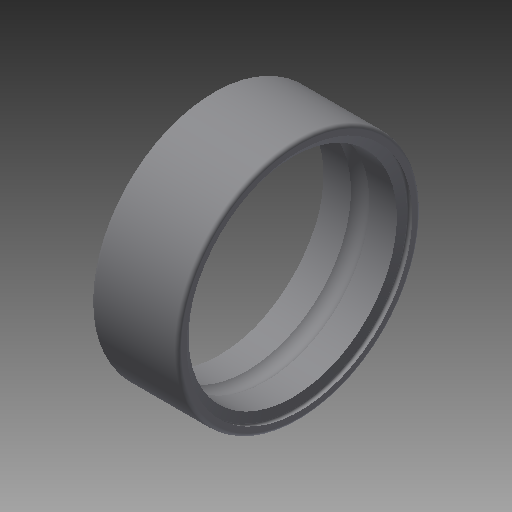
# Autodesk Inventor part: W 627/4-2Z_PART2
Saved by Autodesk Inventor 2018.3 (Build 223284000, 284)
## iProperties
Category: PARTsolutions
Company: SKF
Created: 2018-07-21
Part Number: W 627/4-2Z_PART2
Material: Generic
Catalog Web Link: www.cadenas.de
Description: -Deep groove ball bearings, stainless steel, single row
Vendor: SKF
Document SubType Name: Modeling
Designer: psadmin
Manufacturer: SKF
Mass: 0.02282 g
Surface Area: 1.23639 cm^2
Volume: 0.02282 cm^3
Density: 1 g/cm^3
Appearance: PSOLRGB-175-175-175
PSOL_IDENT_0: {$CADENAS_DATA\23d-libs\skf\bearings_units_and_housings\ball_bearings\deep_groove_ball_bearings\deep
PSOL_IDENT_1: _groove_ball_bearings_stainless_steel\bb1_004_104.prj},199 {VTYP=3D},{NB=W 627/4-2Z_PART2},{LINA=W 6
PSOL_IDENT_2: 27/4-2Z_PART2},{NN=BB1_004_104_PART2},{NOPRJ=TRUE},{DATE=13.07.2018 14:28:03},{GEOMDATE=26.07.2017 1
PSOL_IDENT_3: 2:34:56},{VERSION=},{LINEID=77220},{WBVAR=},{WBNUMERIC=}  {NB=W 627/4-2Z_PART2},{LINA=W 627/4-2Z_PAR
PSOL_IDENT_4: T2},{KT=DUMMY},{PRODUCTID=},{DESIGNATION=W 627/4-2Z},{DD=4.000},{D=7.000},{B=2.500},{DD1=4.800},{DD2=
PSOL_IDENT_5: MIN},{D1=6.000},{D2=6.500},{R12A=0.100},{LOAD1=0.143},{LOAD2=0.053},{LOAD3=0.002},{SPEED1=75000},{SP
PSOL_IDENT_6: EED2=},{MASS=0.000},{PITCH=5.400},{DW=0.800},{Z=11.000},{II=1.000},{TYPEID=MIN},{YALG=2.4},{HALG=0.4
PSOL_IDENT_7: },{HELP=0.5},{HELP2=0.25},{YALG1=3},{HALG1=0.5},{TAXONOMY=2},{DESIGN=dgbbw2z},{MAPPING=BCZ50,DESIGNA
PSOL_IDENT_8: TION|IRD01,DD|ORD10,D|BCW30,B|IRD30,DD1|ORD30,D1|ORD43,D2|IRD43,DD2|ORR20,R12A|BCC02,LOAD1|BCC16,LOA
PSOL_IDENT_9: D2|BCC12,LOAD3|BCC45,SPEED1|BCM01,MASS|BCD50,PITCH|RBD10,DW|BCN81,Z|BCN80,II},{DESIGNLIST=dgbbw2z,dg
PSOL_IDENT_10: bbw,dgbbw2rs},{SH=2.4},{SORT=DD},{RHELP=0.1},{PIM=W 627/4-2Z},{R12=0.1},{HIDE=MIN}
NT: Deep groove ball bearings, stainless steel, single row
NB: W 627/4-2Z_PART2
NBSYN: $DESIGNATION._PART2
LINA: W 627/4-2Z_PART2
SUPPLIER: SKF
ARTICLENO: W 627/4-2Z_PART2
BOMINFO: W 627/4-2Z_PART2
CREATOR: CADENAS GmbH
Title: W 627/4-2Z_PART2
Author: Cadenas PARTsolutions
Comments: Deep groove ball bearings, stainless steel, single row
Autodesk Inventor part; units mm, degrees
ref_plane "YZ Plane" through (0, 0, 0) normal (1, 0, 0) x (0, 1, 0)
ref_plane "XZ Plane" through (0, 0, 0) normal (0, 1, 0) x (-1, 0, 0)
ref_plane "XY Plane" through (0, 0, 0) normal (0, 0, 1) x (1, 0, 0)
sketch "Sketch_6" plane through (0, 0, 0) normal (0, 0, 1) x (1, 0, 0)
  line L0 (50, 0) -> (-50, 0)
  line L1 (0, 3.4) -> (0, 3.25)
  line L2 (0, 3.25) -> (0.03, 3.25)
  arc A0 (0.15, 3.25) -> (0.03, 3.25) centre (0.09, 3.25) ccw
  line L3 (0.15, 3.25) -> (0.1941, 3)
  line L4 (0.1941, 3) -> (0.9854, 3)
  arc A1 (1.5146, 3) -> (0.9854, 3) centre (1.25, 2.7) ccw
  line L5 (1.5146, 3) -> (2.3059, 3)
  line L6 (2.3059, 3) -> (2.35, 3.25)
  arc A2 (2.47, 3.25) -> (2.35, 3.25) centre (2.41, 3.25) ccw
  line L7 (2.47, 3.25) -> (2.5, 3.25)
  line L8 (2.5, 3.25) -> (2.5, 3.4)
  arc A3 (2.5, 3.4) -> (2.4, 3.5) centre (2.4, 3.4) ccw
  line L9 (2.4, 3.5) -> (0.1, 3.5)
  arc A4 (0.1, 3.5) -> (0, 3.4) centre (0.1, 3.4) ccw
  constraints: 20 end point, 10 point on circle, 5 centre point
revolve "Revolution1" add sketch "Sketch_6" angle 360 about axis through (50, 0, 0) along (1, 0, 0)
body "Solid1"
